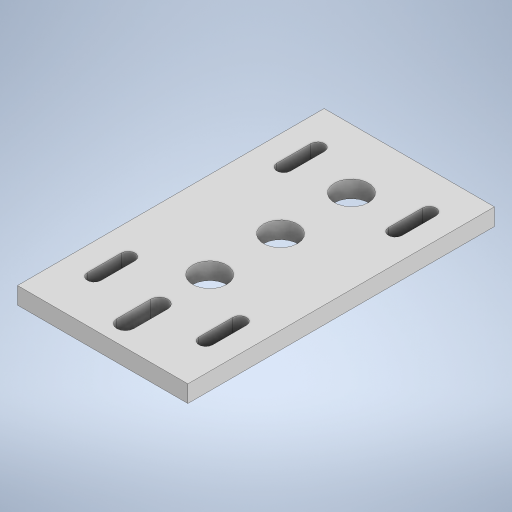
# Autodesk Inventor part: Sliding Plate
Saved by Autodesk Inventor 2023 (Build 270158000, 158)
## iProperties
Created: 2022-06-19
Part Number: Sliding Plate
Material: Generic
Document SubType Name: Modeling
Designer: Shivan
Density: 1 g/cm^3
Appearance: Default
Author: Shivan
Autodesk Inventor part; units mm, degrees
ref_plane "YZ Plane" through (0, 0, 0) normal (1, 0, 0) x (0, 1, 0)
ref_plane "XZ Plane" through (0, 0, 0) normal (0, 1, 0) x (-1, 0, 0)
ref_plane "XY Plane" through (0, 0, 0) normal (0, 0, 1) x (1, 0, 0)
sketch "Sketch1" plane through (0, 0, 0) normal (0, 1, 0) x (-1, 0, 0)
  line L0 (0, 0) -> (100, 0)
  line L1 (100, 0) -> (100, -180)
  line L2 (100, -180) -> (0, -180)
  line L3 (0, -180) -> (0, 0)
  dimension "d0" = 100
  dimension "d1" = 180
  constraints: 8 end point, 2 parallel, 1 horizontal, 1 perpendicular
  measures "d0" distance of L1.end L2.end
  measures "d1" distance of L0.end L1.end
sketch "Sketch2" plane through (0, 0, 0) normal (0, 1, 0) x (-1, 0, 0)
  circle A0 centre (49.0743, -61.8964) radius 10
  circle A1 centre (49.0743, -103.4918) radius 10
  circle A2 centre (49.0743, -145.129) radius 10
  line L0 (82.079, -27.0534) -> (82.079, -47.0534) construction
  line L1 (86.0942, -27.0534) -> (86.0942, -47.0534)
  line L2 (78.0638, -47.0534) -> (78.0638, -27.0534)
  arc A3 (86.0942, -27.0534) -> (78.0638, -27.0534) centre (82.079, -27.0534) ccw
  arc A4 (78.0638, -47.0534) -> (86.0942, -47.0534) centre (82.079, -47.0534) ccw
  line L3 (16.5655, -27.0534) -> (16.5655, -47.0534) construction
  line L4 (20.5808, -27.0534) -> (20.5808, -47.0534)
  line L5 (12.5503, -47.0534) -> (12.5503, -27.0534)
  arc A5 (20.5808, -27.0534) -> (12.5503, -27.0534) centre (16.5655, -27.0534) ccw
  arc A6 (12.5503, -47.0534) -> (20.5808, -47.0534) centre (16.5655, -47.0534) ccw
  line L6 (82.079, -138.3165) -> (82.079, -158.3165) construction
  line L7 (86.0942, -138.3165) -> (86.0942, -158.3165)
  line L8 (78.0638, -158.3165) -> (78.0638, -138.3165)
  arc A7 (86.0942, -138.3165) -> (78.0638, -138.3165) centre (82.079, -138.3165) ccw
  arc A8 (78.0638, -158.3165) -> (86.0942, -158.3165) centre (82.079, -158.3165) ccw
  line L9 (16.5655, -138.3165) -> (16.5655, -158.3165) construction
  line L10 (20.5808, -138.3165) -> (20.5808, -158.3165)
  line L11 (12.5503, -158.3165) -> (12.5503, -138.3165)
  arc A9 (20.5808, -138.3165) -> (12.5503, -138.3165) centre (16.5655, -138.3165) ccw
  arc A10 (12.5503, -158.3165) -> (20.5808, -158.3165) centre (16.5655, -158.3165) ccw
  point P0 (0, 0)
  point P1 (82.079, -37.0534)
  point P2 (16.5655, -37.0534)
  point P3 (82.079, -148.3165)
  point P4 (16.5655, -148.3165)
  dimension "d3" = 20
  dimension "d13" = 20
  dimension "d14" = 20
  dimension "d15" = 20
  dimension "d16" = 20
  constraints: 32 end point, 16 point on circle, 16 tangent, 11 centre point, 4 midpoint, 4 parallel, 4 vertical
  measures "d3" diameter of A1
  measures "d13" distance of L6.start L6.end
  measures "d14" distance of L9.start L9.end
  measures "d15" distance of L0.start L0.end
  measures "d16" distance of L3.start L3.end
extrude "Extrusion1" add sketch "Sketch1" along normal blind 10
extrude "Extrusion2" cut sketch "Sketch2" along normal blind 10
sketch "Sketch6" plane through (0, 10, 0) normal (0, 1, 0) x (1, 0, 0)
  line L0 (-48.9569, 12.2049) -> (-48.9569, 32.2049) construction
  line L1 (-43.9569, 12.2049) -> (-43.9569, 32.2049)
  line L2 (-53.9569, 32.2049) -> (-53.9569, 12.2049)
  arc A0 (-53.9569, 12.2049) -> (-43.9569, 12.2049) centre (-48.9569, 12.2049) ccw
  arc A1 (-43.9569, 32.2049) -> (-53.9569, 32.2049) centre (-48.9569, 32.2049) ccw
  point P0 (0, 0)
  point P1 (-48.9569, 22.2049)
  dimension "d9" = 20
  constraints: 8 end point, 4 point on circle, 4 tangent, 2 centre point, 1 midpoint, 1 parallel, 1 vertical
  measures "d9" distance of L0.start L0.end
extrude "Extrusion3" cut sketch "Sketch6" against normal blind 10
body "Solid1"
